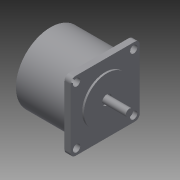
# Autodesk Inventor part: Pieza27
Saved by Autodesk Inventor 2015 (Build 190159000, 159)
## iProperties
Created: 2015-02-17
Part Number: Pieza27
Material: Genérico
Document SubType Name: Modeling
Designer: jorge
Density: 1 g/cm^3
Appearance: Valor por defecto
Author: jorge
Autodesk Inventor part; units mm, degrees
ref_plane "YZ Plane" through (0, 0, 0) normal (1, 0, 0) x (0, 1, 0)
ref_plane "XZ Plane" through (0, 0, 0) normal (0, 1, 0) x (-1, 0, 0)
ref_plane "XY Plane" through (0, 0, 0) normal (0, 0, 1) x (1, 0, 0)
sketch "Boceto1" plane through (0, 0, 0) normal (1, 0, 0) x (0, 1, 0)
  circle A0 centre (0, 0) radius 28.5
  dimension "d0" = 57
  constraints: 1 centre point, 1 coincident
  measures "d0" diameter of A0
extrude "cuerpo" add sketch "Boceto1" along normal blind 40
sketch "Boceto2" plane through (40, 0, 0) normal (1, 0, 0) x (0, 0, -1)
  line L0 (-24.5, 28.5) -> (24.5, 28.5)
  line L1 (28.5, 24.5) -> (28.5, -24.5)
  line L2 (24.5, -28.5) -> (-24.5, -28.5)
  line L3 (-28.5, -24.5) -> (-28.5, 24.5)
  line L4 (-28.5, 28.5) -> (28.5, -28.5) construction
  line L5 (28.5, 28.5) -> (-28.5, -28.5) construction
  arc A0 (28.5, 24.5) -> (24.5, 28.5) centre (24.5, 24.5) ccw
  arc A1 (-24.5, 28.5) -> (-28.5, 24.5) centre (-24.5, 24.5) ccw
  arc A2 (-28.5, -24.5) -> (-24.5, -28.5) centre (-24.5, -24.5) ccw
  arc A3 (24.5, -28.5) -> (28.5, -24.5) centre (24.5, -24.5) ccw
  point P0 (0, 0)
  dimension "d3" = 57
  dimension "d4" = 57
  dimension "d16" = 4
  constraints: 12 end point, 8 point on circle, 8 point on line, 8 tangent, 4 centre point, 3 equal radius, 2 midpoint, 2 parallel, 1 horizontal, 1 perpendicular
  measures "d3" distance of L4.end L5.end
  measures "d4" distance of L5.start L4.end
  measures "d16" radius of A0
extrude "cara" add sketch "Boceto2" along normal blind 5
sketch "Boceto3" plane through (45, 0, 0) normal (1, 0, 0) x (0, 0, -1)
  circle A0 centre (0, 0) radius 19
  dimension "d7" = 38
  constraints: 1 centre point, 1 coincident
  measures "d7" diameter of A0
extrude "Extrusión3" add sketch "Boceto3" along normal blind 1.5
sketch "Boceto4" plane through (46.5, 0, 0) normal (1, 0, 0) x (0, 0, -1)
  circle A0 centre (0, 0) radius 4
  dimension "d10" = 8
  constraints: 1 centre point, 1 coincident
  measures "d10" diameter of A0
extrude "Extrusión4" cut sketch "Boceto4" against normal blind 1.5
sketch "Boceto5" plane through (45, 0, 0) normal (1, 0, 0) x (0, 0, -1)
  circle A0 centre (0, 0) radius 3
  dimension "d13" = 6
  constraints: 1 centre point, 1 coincident
  measures "d13" diameter of A0
extrude "Extrusión5" add sketch "Boceto5" along normal blind 20
sketch "Boceto6" plane through (45, 0, 0) normal (1, 0, 0) x (0, 0, -1)
  line L0 (24.5, 28.5) -> (-24.5, 28.5) projected
  line L1 (-28.5, 24.5) -> (-28.5, -24.5) projected
  line L2 (-28.5, 0) -> (28.2081, 0)
  line L3 (0, 28.5) -> (0, -28.5)
  line L4 (-24.5, -28.5) -> (24.5, -28.5) projected
  line L5 (-24.5, -28.5) -> (-23.5, -28.5)
  line L6 (0, -28.5) -> (-24.5, -28.5) projected
  line L7 (-23.5, -28.5) -> (-23.5, -23.5)
  circle A0 centre (-23.5, -23.5) radius 3
  circle A1 centre (23.5, -23.5) radius 3
  circle A2 centre (-23.5, 23.5) radius 3
  circle A3 centre (23.5, 23.5) radius 3
  point P0 (0, 0)
  dimension "d22" = 1
  dimension "d23" = 5
  dimension "d24" = 6
  constraints: 8 end point, 4 centre point, 3 midpoint, 3 symmetric about line, 1 coincident, 1 horizontal, 1 perpendicular, 1 point on line, 3 other
  measures "d22" distance of L4.start L5.end
  measures "d23" distance of L5.end L7.end
  measures "d24" diameter of A0
extrude "Extrusión6" cut sketch "Boceto6" against normal up to surface (5 mm away)
